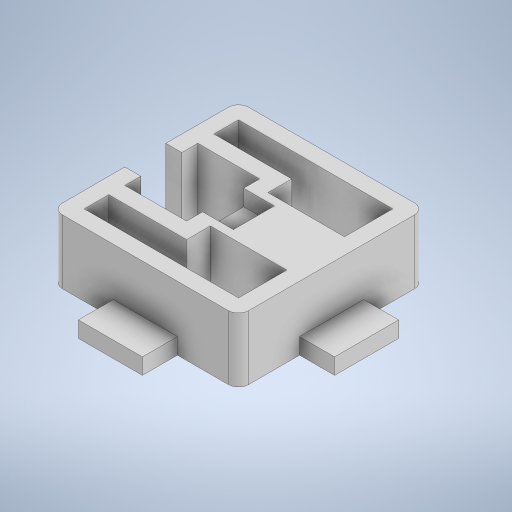
# Autodesk Inventor part: hall holder
Saved by Autodesk Inventor 2024 (Build 280153000, 153)
## iProperties
Created: 2024-04-10
Part Number: hall holder
Material: Generic
Document SubType Name: Modeling
Designer: drew
Density: 1 g/cm^3
Appearance: Default
Author: drew
Autodesk Inventor part; units mm, degrees
ref_plane "YZ Plane" through (0, 0, 0) normal (1, 0, 0) x (0, 1, 0)
ref_plane "XZ Plane" through (0, 0, 0) normal (0, 1, 0) x (-1, 0, 0)
ref_plane "XY Plane" through (0, 0, 0) normal (0, 0, 1) x (1, 0, 0)
sketch "Sketch1" plane through (0, 0, 0) normal (0, 1, 0) x (-1, 0, 0)
  line L0 (-9.2329, 9.2329) -> (9.2329, 9.2329)
  line L1 (9.2329, -9.2329) -> (-9.2329, -9.2329)
  line L2 (-9.2329, -9.2329) -> (-9.2329, 9.2329)
  line L3 (-9.2329, 9.2329) -> (9.2329, -9.2329) construction
  line L4 (9.2329, 9.2329) -> (-9.2329, -9.2329) construction
  line L5 (-1.524, 2.032) -> (1.524, 2.032) construction
  line L6 (1.524, 2.032) -> (1.524, -2.032) construction
  line L7 (1.524, -2.032) -> (-1.524, -2.032) construction
  line L8 (-1.524, -2.032) -> (-1.524, 2.032) construction
  line L9 (-1.524, 2.032) -> (1.524, -2.032) construction
  line L10 (1.524, 2.032) -> (-1.524, -2.032) construction
  line L11 (1.524, 2.032) -> (9.2329, 2.032)
  line L12 (9.2329, -2.032) -> (1.524, -2.032)
  line L13 (1.524, -2.032) -> (1.524, 2.032)
  line L14 (9.2329, 9.2329) -> (9.2329, 2.032)
  line L15 (9.2329, -2.032) -> (9.2329, -9.2329)
  point P0 (0, 0)
  dimension "d0" = 18.4658
  dimension "d1" = 3.048
  dimension "d2" = 4.064
  constraints: 32 end point, 6 parallel, 4 midpoint, 4 perpendicular, 3 horizontal, 1 collinear
  measures "d0" distance of L1.start L1.end
  measures "d1" distance of L6.end L7.end
  measures "d2" distance of L7.end L5.start
extrude "Extrusion1" add sketch "Sketch1" along normal blind 6.35
sketch "Sketch2" plane through (-1.524, 0, -2.032) normal (-1, 0, 0) x (0, 0, 1)
  line L0 (0, 0) -> (4.064, 0) projected
  line L1 (4.064, 0) -> (4.064, 6.35) projected
  line L2 (0, 6.35) -> (4.064, 6.35) projected
  line L3 (0, 0) -> (0, 6.35) projected
  line L4 (0, 4.7498) -> (4.064, 4.7498)
  line L5 (0, 5.5118) -> (0.762, 6.35)
  line L6 (3.302, 6.35) -> (4.064, 5.5118)
  line L7 (2.032, 4.7498) -> (2.032, 6.35) construction
  point P0 (2.032, 0)
  dimension "d17" = 1.6002
  dimension "d19" = 2.54
  dimension "d21" = 0.762
  constraints: 8 end point, 7 point on line, 2 midpoint, 1 horizontal alignment, 1 perpendicular, 1 other
  measures "d17" distance between parallel lines of L2 L4
  measures "d19" distance of L6.start L5.end
  measures "d21" distance from line of L4 L5.start
extrude "Extrusion2" cut sketch "Sketch2" against normal blind 3.048 contours L3 L5 L2 L6 L1 L4
sketch "Sketch6" plane through (0, 6.35, 0) normal (0, 1, 0) x (1, 0, 0)
  line L0 (1.524, -1.27) -> (-1.524, -1.27) projected
  line L1 (-1.524, -1.27) -> (-1.524, -2.032) projected
  line L2 (-1.524, -2.032) -> (-9.2329, -2.032) projected
  line L3 (-9.2329, -2.032) -> (-9.2329, -9.2329) projected
  line L4 (-9.2329, -9.2329) -> (9.2329, -9.2329) projected
  line L5 (9.2329, -9.2329) -> (9.2329, 9.2329) projected
  line L6 (9.2329, 9.2329) -> (-9.2329, 9.2329) projected
  line L7 (-9.2329, 9.2329) -> (-9.2329, 2.032) projected
  line L8 (-9.2329, 2.032) -> (-1.524, 2.032) projected
  line L9 (-1.524, 2.032) -> (-1.524, 1.27) projected
  line L10 (-1.524, 1.27) -> (1.524, 1.27) projected
  line L11 (1.524, 1.27) -> (1.524, -1.27) projected
  line L12 (-7.6454, 7.6454) -> (7.6454, 7.6454)
  line L13 (7.6454, 7.6454) -> (7.6454, -7.6454)
  line L14 (7.6454, -7.6454) -> (-7.6454, -7.6454)
  line L15 (-7.6454, -7.6454) -> (-7.6454, -3.6195)
  line L16 (-7.6454, -3.6195) -> (0.0635, -3.6195)
  line L17 (0.0635, -3.6195) -> (0.0635, -2.8575)
  line L18 (0.0635, -2.8575) -> (3.1115, -2.8575)
  line L19 (3.1115, -2.8575) -> (3.1115, 2.8575)
  line L20 (3.1115, 2.8575) -> (0.0635, 2.8575)
  line L21 (0.0635, 2.8575) -> (0.0635, 3.6195)
  line L22 (0.0635, 3.6195) -> (-7.6454, 3.6195)
  line L23 (-7.6454, 3.6195) -> (-7.6454, 7.6454)
  line L24 (-7.6454, 3.6195) -> (-1.524, 3.6195)
  line L25 (-1.524, 3.6195) -> (-1.524, -3.6195)
  line L26 (-1.524, -3.6195) -> (-7.6454, -3.6195)
  line L27 (-7.6454, -3.6195) -> (-7.6454, 3.6195)
  point P0 (0, 0)
  point P1 (-7.6454, -2.032)
  point P2 (-7.6454, 2.032)
  point P3 (-1.524, 2.032)
  dimension "d22" = 1.5875
  constraints: 32 end point, 2 parallel, 1 collinear, 1 horizontal, 1 perpendicular, 1 point on line, 11 other
  measures "d22" distance between parallel lines of L6 L12
extrude "Extrusion5" cut sketch "Sketch6" against normal through all contours L25 L16 L27 L2 | L8 L27 L22 L25
sketch "Sketch7" plane through (0, 6.35, 0) normal (0, 1, 0) x (1, 0, 0)
  line L0 (-7.6454, -3.6195) -> (-7.6454, -2.032) projected
  line L1 (-7.6454, -2.032) -> (-9.2329, -2.032) projected
  line L2 (-9.2329, -2.032) -> (-9.2329, -9.2329) projected
  line L3 (-9.2329, -9.2329) -> (9.2329, -9.2329) projected
  line L4 (9.2329, -9.2329) -> (9.2329, 9.2329) projected
  line L5 (9.2329, 9.2329) -> (-9.2329, 9.2329) projected
  line L6 (-9.2329, 9.2329) -> (-9.2329, 2.032) projected
  line L7 (-9.2329, 2.032) -> (-7.6454, 2.032) projected
  line L8 (-7.6454, 2.032) -> (-7.6454, 3.6195) projected
  line L9 (-7.6454, 3.6195) -> (-1.524, 3.6195) projected
  line L10 (-1.524, 3.6195) -> (-1.524, 1.27) projected
  line L11 (-1.524, 1.27) -> (1.524, 1.27) projected
  line L12 (1.524, 1.27) -> (1.524, -1.27) projected
  line L13 (1.524, -1.27) -> (-1.524, -1.27) projected
  line L14 (-1.524, -1.27) -> (-1.524, -3.6195) projected
  line L15 (-1.524, -3.6195) -> (-7.6454, -3.6195) projected
  line L16 (-7.6454, 7.6454) -> (7.6454, 7.6454)
  line L17 (7.6454, 7.6454) -> (7.6454, -7.6454)
  line L18 (7.6454, -7.6454) -> (-7.6454, -7.6454)
  line L19 (-7.6454, -7.6454) -> (-7.6454, -5.207)
  line L20 (-7.6454, -5.207) -> (0.0635, -5.207)
  line L21 (0.0635, -5.207) -> (0.0635, -2.8575)
  line L22 (0.0635, -2.8575) -> (3.1115, -2.8575)
  line L23 (3.1115, -2.8575) -> (3.1115, 2.8575)
  line L24 (3.1115, 2.8575) -> (0.0635, 2.8575)
  line L25 (0.0635, 2.8575) -> (0.0635, 5.207)
  line L26 (0.0635, 5.207) -> (-7.6454, 5.207)
  line L27 (-7.6454, 5.207) -> (-7.6454, 7.6454)
  point P0 (0, 0)
  dimension "d25" = 1.5875
  constraints: 24 end point, 11 other
  measures "d25" distance between parallel lines of L5 L16
extrude "Extrusion6" cut sketch "Sketch7" against normal through all contours L16 L17 L18 L19 L20 L21 L22 L23 L24 L25 L26 L27
sketch "Sketch8" plane through (0, 0, 0) normal (0, -1, 0) x (1, 0, 0)
  line L0 (-3.175, -12.7) -> (3.175, -12.7)
  line L1 (3.175, -12.7) -> (3.175, 12.7)
  line L2 (3.175, 12.7) -> (-3.175, 12.7)
  line L3 (-3.175, 12.7) -> (-3.175, -12.7)
  line L4 (-3.175, -12.7) -> (3.175, 12.7) construction
  line L5 (3.175, -12.7) -> (-3.175, 12.7) construction
  line L6 (0.0635, -5.207) -> (0.0635, -2.8575) projected
  line L7 (0.0635, -2.8575) -> (3.1115, -2.8575) projected
  line L8 (3.1115, -2.8575) -> (3.1115, 2.8575) projected
  line L9 (3.1115, 2.8575) -> (0.0635, 2.8575) projected
  line L10 (0.0635, 2.8575) -> (0.0635, 5.207) projected
  line L11 (0.0635, 5.207) -> (-7.6454, 5.207) projected
  line L12 (-7.6454, 5.207) -> (-7.6454, 7.6454) projected
  line L13 (-7.6454, 7.6454) -> (7.6454, 7.6454) projected
  line L14 (7.6454, 7.6454) -> (7.6454, -7.6454) projected
  line L15 (7.6454, -7.6454) -> (-7.6454, -7.6454) projected
  line L16 (-7.6454, -7.6454) -> (-7.6454, -5.207) projected
  line L17 (-7.6454, -5.207) -> (0.0635, -5.207) projected
  line L18 (-7.6454, 2.032) -> (-7.6454, 3.6195) projected
  line L19 (-7.6454, 3.6195) -> (-1.524, 3.6195) projected
  line L20 (-1.524, -3.6195) -> (-1.524, 3.6195) projected
  line L21 (-1.524, -3.6195) -> (-7.6454, -3.6195) projected
  line L22 (-7.6454, -3.6195) -> (-7.6454, -2.032) projected
  line L23 (-9.2329, -2.032) -> (-7.6454, -2.032) projected
  line L24 (-9.2329, -9.2329) -> (-9.2329, -2.032) projected
  line L25 (9.2329, -9.2329) -> (-9.2329, -9.2329) projected
  line L26 (9.2329, 9.2329) -> (9.2329, -9.2329) projected
  line L27 (-9.2329, 9.2329) -> (9.2329, 9.2329) projected
  line L28 (-9.2329, 2.032) -> (-9.2329, 9.2329) projected
  line L29 (-7.6454, 2.032) -> (-9.2329, 2.032) projected
  line L30 (-12.7, 3.175) -> (-12.7, -3.175)
  line L31 (-12.7, -3.175) -> (12.7, -3.175)
  line L32 (12.7, -3.175) -> (12.7, 3.175)
  line L33 (12.7, 3.175) -> (-12.7, 3.175)
  point P0 (0, 0)
  point P1 (3.175, -9.2329)
  point P2 (-3.175, -9.2329)
  point P3 (9.2329, 3.175)
  point P4 (9.2329, -3.175)
  point P5 (-3.175, 9.2329)
  point P6 (3.175, 9.2329)
  dimension "d28" = 6.35
  dimension "d29" = 25.4
  dimension "d32" = 90
  constraints: 20 end point, 2 midpoint, 2 parallel, 1 horizontal, 1 perpendicular, 9 other
  measures "d28" distance of L1.end L2.end
  measures "d29" distance of L2.end L0.start
extrude "Extrusion7" add sketch "Sketch8" against normal blind 1.5875 contours L3 L25 L1 L0 | L26 L33 L32 L31 | L27 L3 L2 L1
sketch "Sketch9" plane through (0, 0, 0) normal (0, -1, 0) x (1, 0, 0)
  line L0 (-1.524, -2.032) -> (1.524, -2.032) projected
  line L1 (0.0635, -5.207) -> (0.0635, -2.8575) projected
  line L2 (0.0635, -2.8575) -> (3.1115, -2.8575) projected
  line L3 (3.1115, -2.8575) -> (3.1115, 2.8575) projected
  line L4 (3.1115, 2.8575) -> (0.0635, 2.8575) projected
  line L5 (0.0635, 2.8575) -> (0.0635, 5.207) projected
  line L6 (0.0635, 5.207) -> (-7.6454, 5.207) projected
  line L7 (-7.6454, 5.207) -> (-7.6454, 7.6454) projected
  line L8 (-7.6454, 7.6454) -> (7.6454, 7.6454) projected
  line L9 (7.6454, 7.6454) -> (7.6454, -7.6454) projected
  line L10 (7.6454, -7.6454) -> (-7.6454, -7.6454) projected
  line L11 (-7.6454, -7.6454) -> (-7.6454, -5.207) projected
  line L12 (-7.6454, -5.207) -> (0.0635, -5.207) projected
  line L13 (-7.6454, 2.032) -> (-7.6454, 3.6195) projected
  line L14 (-7.6454, 3.6195) -> (-1.524, 3.6195) projected
  line L15 (-1.524, -3.6195) -> (-1.524, 3.6195) projected
  line L16 (-1.524, -3.6195) -> (-7.6454, -3.6195) projected
  line L17 (-7.6454, -3.6195) -> (-7.6454, -2.032) projected
  line L18 (-9.2329, -2.032) -> (-7.6454, -2.032) projected
  line L19 (-9.2329, -9.2329) -> (-9.2329, -2.032) projected
  line L20 (-3.175, -9.2329) -> (-9.2329, -9.2329) projected
  line L21 (-3.175, -9.2329) -> (-3.175, -12.7) projected
  line L22 (-3.175, -12.7) -> (3.175, -12.7) projected
  line L23 (3.175, -12.7) -> (3.175, -9.2329) projected
  line L24 (9.2329, -9.2329) -> (3.175, -9.2329) projected
  line L25 (9.2329, -3.175) -> (9.2329, -9.2329) projected
  line L26 (9.2329, -3.175) -> (12.7, -3.175) projected
  line L27 (12.7, -3.175) -> (12.7, 3.175) projected
  line L28 (12.7, 3.175) -> (9.2329, 3.175) projected
  line L29 (9.2329, 9.2329) -> (9.2329, 3.175) projected
  line L30 (3.175, 9.2329) -> (9.2329, 9.2329) projected
  line L31 (3.175, 9.2329) -> (3.175, 12.7) projected
  line L32 (3.175, 12.7) -> (-3.175, 12.7) projected
  line L33 (-3.175, 12.7) -> (-3.175, 9.2329) projected
  line L34 (-9.2329, 9.2329) -> (-3.175, 9.2329) projected
  line L35 (-9.2329, 2.032) -> (-9.2329, 9.2329) projected
  line L36 (-7.6454, 2.032) -> (-9.2329, 2.032) projected
  line L37 (3.1115, -2.8575) -> (7.6454, -2.8575)
  line L38 (7.6454, -2.8575) -> (7.6454, 2.8575)
  line L39 (7.6454, 2.8575) -> (3.1115, 2.8575)
  line L40 (3.1115, 2.8575) -> (3.1115, -2.8575)
  line L41 (3.1115, 2.8575) -> (0.0635, 2.8575) projected
  point P0 (0, 0)
  point P1 (7.6454, 2.8575)
  constraints: 8 end point, 2 collinear, 2 parallel, 1 horizontal, 1 perpendicular
extrude "Extrusion8" add sketch "Sketch9" against normal up to surface (6.35 mm away) contours L3 L39 L9 L37
sketch "Sketch10" plane through (-1.524, 4.7498, 2.032) normal (-1, 0, 0) x (0, 0, 1)
  line L0 (-0.762, 1.6002) -> (0, 0.762) projected
  line L1 (0, 0) -> (0, 0.762) projected
  line L2 (0, 0) -> (-4.064, 0) projected
  line L3 (-4.064, 0.762) -> (-4.064, 0) projected
  line L4 (-4.064, 0.762) -> (-3.302, 1.6002) projected
  line L5 (-5.6515, 1.6002) -> (-3.302, 1.6002) projected
  line L6 (-5.6515, 1.6002) -> (-5.6515, -4.7498) projected
  line L7 (-5.6515, -4.7498) -> (1.5875, -4.7498) projected
  line L8 (1.5875, 1.6002) -> (1.5875, -4.7498) projected
  line L9 (-0.762, 1.6002) -> (1.5875, 1.6002) projected
  line L10 (-11.2649, -4.7498) -> (-4.064, -4.7498) projected
  line L11 (-4.064, -4.7498) -> (-4.064, 1.6002) projected
  line L12 (-11.2649, 1.6002) -> (-4.064, 1.6002) projected
  line L13 (-11.2649, -4.7498) -> (-11.2649, 1.6002) projected
  line L14 (0, -4.7498) -> (7.2009, -4.7498) projected
  line L15 (7.2009, -4.7498) -> (7.2009, 1.6002) projected
  line L16 (0, 1.6002) -> (7.2009, 1.6002) projected
  line L17 (0, -4.7498) -> (0, 1.6002) projected
  point P0 (-2.032, -4.7498)
extrude "Extrusion9" cut sketch "Sketch10" against normal up to surface (3.048 mm away) contours L9 L17 L0 | L11 L5 L4
fillet "Fillet3" radius 1 4 edges at (-9.2329, 3.175, -9.2329) (-9.2329, 3.175, 9.2329) (9.2329, 3.175, 9.2329) (9.2329, 3.175, -9.2329)
body "Solid1"
